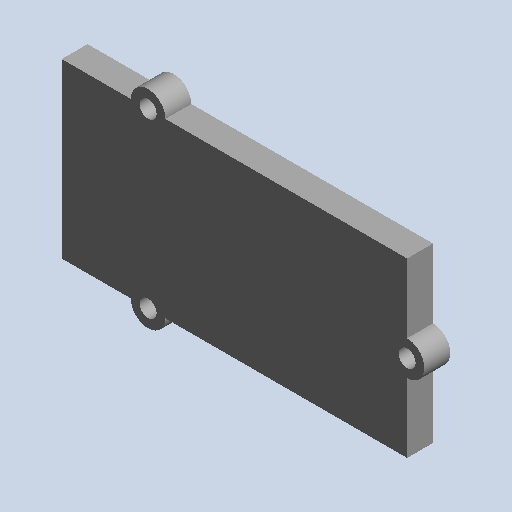
# Autodesk Inventor part: current sensor
Saved by Autodesk Inventor 2026 (Build 300175050, 175E)
## iProperties
Part Number: current sensor
Material: Generic
Document SubType Name: Modeling
Designer: Kartik
Mass: 2.42827 g
Surface Area: 20.5595 cm^2
Volume: 2.42827 cm^3
Density: 1 g/cm^3
Appearance: Default
Author: Kartik
Autodesk Inventor part; units mm, degrees
ref_plane "YZ Plane" through (0, 0, 0) normal (1, 0, 0) x (0, 1, 0)
ref_plane "XZ Plane" through (0, 0, 0) normal (0, 1, 0) x (-1, 0, 0)
ref_plane "XY Plane" through (0, 0, 0) normal (0, 0, 1) x (1, 0, 0)
sketch "Sketch1" plane through (0, 0, 0) normal (0, 0, 1) x (1, 0, 0)
  line L0 (-20, -10) -> (-20, 10)
  circle A0 centre (20, 0) radius 1
  arc A1 (20, -2) -> (20, 2) centre (20, 0) ccw
  line L1 (20, 10) -> (20, 2)
  line L2 (20, -2) -> (20, -10)
  circle A2 centre (-10, -10) radius 1
  arc A3 (-12, -10) -> (-8, -10) centre (-10, -10) ccw
  circle A4 centre (-10, 10) radius 1
  arc A5 (-8, 10) -> (-12, 10) centre (-10, 10) ccw
  line L3 (20, -10) -> (-8, -10)
  line L4 (-12, -10) -> (-20, -10)
  line L5 (-10, -10) -> (-9, -10)
  line L6 (-8, -10) -> (20, -10)
  line L7 (-20, 10) -> (-12, 10)
  line L8 (-8, 10) -> (20, 10)
  point P0 (0, 0)
  dimension "d8" = 2
  dimension "d0" = 20
  dimension "d1" = 40
  dimension "d4" = 2
  dimension "d5" = 4
  dimension "d6" = 0
  dimension "d7" = 10
  dimension "d9" = 4
  dimension "d10" = 2
  dimension "d11" = 4
  constraints: 18 end point, 6 parallel, 6 point on circle, 5 centre point, 4 coincident, 4 collinear, 4 perpendicular, 2 horizontal, 1 horizontal alignment, 2 other
  measures "d0" distance of L0.start L0.end
  measures "d1" distance of L0.end L1.start
  measures "d4" diameter of A0
  measures "d5" diameter of A1
  measures "d6" vertical distance of point (0, 0) A0.centre
  measures "d7" distance from line of L0 L5.start
  measures "d9" diameter of A3
  measures "d10" diameter of A4
  measures "d11" diameter of A5
extrude "Extrusion1" add sketch "Sketch1" along normal blind 3
body "Solid1"
